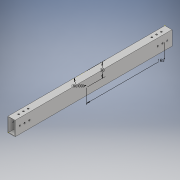
# Autodesk Inventor part: nhk39
Saved by Autodesk Inventor 2019 (Build 230136000, 136)
## iProperties
Created: 2022-02-27
Part Number: nhk39
Material: 一般
Document SubType Name: Sheet Metal
Designer: yuta
Density: 1 g/cm^3
Sheet Metal Rule: Default_mm
Appearance: 既定
Author: yuta
Autodesk Inventor part; units mm, degrees
ref_plane "YZ Plane" through (0, 0, 0) normal (1, 0, 0) x (0, 1, 0)
ref_plane "XZ Plane" through (0, 0, 0) normal (0, 1, 0) x (-1, 0, 0)
ref_plane "XY Plane" through (0, 0, 0) normal (0, 0, 1) x (1, 0, 0)
sketch "スケッチ1" plane through (0, 0, 0) normal (0, 0, 1) x (1, 0, 0)
  line L0 (0, 0) -> (15, 0)
  line L1 (15, 0) -> (15, 30)
  line L2 (15, 30) -> (0, 30)
  line L3 (0, 30) -> (0, 0)
  line L4 (1, 1) -> (14, 1)
  line L5 (14, 1) -> (14, 29)
  line L6 (14, 29) -> (1, 29)
  line L7 (1, 29) -> (1, 1)
  dimension "d0" = 15
  dimension "d1" = 30
  dimension "d2" = 13
  dimension "d3" = 28
  dimension "d4" = 1
  dimension "d5" = 1
  constraints: 16 end point, 4 parallel, 2 horizontal, 2 perpendicular
  measures "d0" distance of L2.end L1.end
  measures "d1" distance of L1.end L0.end
  measures "d2" distance of L6.end L5.end
  measures "d3" distance of L5.end L4.end
  measures "d4" distance between parallel lines of L2 L6
  measures "d5" distance between parallel lines of L3 L7
extrude "押し出し1" add sketch "スケッチ1" along normal blind 330
sketch "スケッチ2" plane through (0, 30, 0) normal (0, 1, 0) x (1, 0, 0)
  circle A0 centre (7.5, -15) radius 1.6
  line L0 (0, 0) -> (0, -330) projected
  line L1 (15, 0) -> (0, 0) projected
  circle A1 centre (7.5, -25) radius 1.6
  circle A2 centre (7.5, -35) radius 1.6
  circle A3 centre (7.5, -315) radius 1.6
  line L2 (15, -330) -> (0, -330) projected
  circle A4 centre (7.5, -305) radius 1.6
  circle A5 centre (7.5, -295) radius 1.6
  dimension "d8" = 3.2
  dimension "d9" = 7.5
  dimension "d10" = 15
  dimension "d11" = 3.2
  dimension "d12" = 10
  dimension "d13" = 3.2
  dimension "d14" = 10
  dimension "d15" = 3.2
  dimension "d16" = 15
  dimension "d17" = 7.5
  dimension "d18" = 3.2
  dimension "d19" = 10
  dimension "d20" = 3.2
  dimension "d21" = 10
  constraints: 6 centre point
  measures "d8" diameter of A0
  measures "d9" distance from line of L0 A0.centre
  measures "d10" distance from line of L1 A0.centre
  measures "d11" diameter of A1
  measures "d12" distance of A0.centre A1.centre
  measures "d13" diameter of A2
  measures "d14" distance of A2.centre A1.centre
  measures "d15" diameter of A3
  measures "d16" distance from line of L2 A3.centre
  measures "d17" distance from line of L0 A3.centre
  measures "d18" diameter of A4
  measures "d19" distance of A3.centre A4.centre
  measures "d20" diameter of A5
  measures "d21" distance of A4.centre A5.centre
hole "穴1" at (7.5, 30, 315) at (7.5, 30, 305) at (7.5, 30, 295) at (7.5, 30, 15) at (7.5, 30, 25) at (7.5, 30, 35) direction (0, -1, 0) diameter 3.2 depth 30
sketch "スケッチ3" plane through (0, 0, 0) normal (-1, 0, 0) x (0, 0, 1)
  circle A0 centre (10, 15) radius 1.6
  line L0 (0, 0) -> (330, 0) projected
  line L1 (0, 30) -> (0, 0) projected
  circle A1 centre (20, 15) radius 1.6
  circle A2 centre (30, 15) radius 1.6
  circle A3 centre (320, 15) radius 1.6
  line L2 (330, 30) -> (330, 0) projected
  circle A4 centre (310, 15) radius 1.6
  circle A5 centre (300, 15) radius 1.6
  dimension "d29" = 3.2
  dimension "d30" = 15
  dimension "d31" = 10
  dimension "d32" = 3.2
  dimension "d33" = 3.2
  dimension "d34" = 10
  dimension "d35" = 10
  dimension "d36" = 3.2
  dimension "d37" = 15
  dimension "d38" = 10
  dimension "d39" = 3.2
  dimension "d40" = 3.2
  dimension "d41" = 10
  dimension "d42" = 10
  dimension "d43" = 15
  dimension "d44" = 15
  dimension "d45" = 15
  dimension "d46" = 15
  constraints: 6 centre point
  measures "d29" diameter of A0
  measures "d30" distance from line of L0 A0.centre
  measures "d31" distance from line of L1 A0.centre
  measures "d32" diameter of A1
  measures "d33" diameter of A2
  measures "d34" distance of A0.centre A1.centre
  measures "d35" distance of A1.centre A2.centre
  measures "d36" diameter of A3
  measures "d37" distance from line of L0 A3.centre
  measures "d38" distance from line of L2 A3.centre
  measures "d39" diameter of A4
  measures "d40" diameter of A5
  measures "d41" distance of A4.centre A3.centre
  measures "d42" distance of A5.centre A4.centre
  measures "d43" distance from line of L0 A4.centre
  measures "d44" distance from line of L0 A5.centre
  measures "d45" distance from line of L0 A1.centre
  measures "d46" distance from line of L0 A2.centre
hole "穴2" at (0, 15, 10) at (0, 15, 20) at (0, 15, 30) at (0, 15, 300) at (0, 15, 310) at (0, 15, 320) direction (1, 0, 0) diameter 3.2 depth 15
sketch "スケッチ4" plane through (0, 0, 0) normal (-1, 0, 0) x (0, 0, 1)
  line L0 (165, 29.8281) -> (165, -0.1719) construction
  line L1 (0, 1) -> (330, 1) projected
  line L2 (165, 29.8281) -> (195, 29.8281) construction
  line L3 (0, 30) -> (0, 0) projected
  dimension "d54" = 30
  dimension "d55" = 90
  dimension "d56" = 165
  constraints: 4 end point, 2 perpendicular, 1 horizontal
  measures "d54" distance of L0.start L0.end
  measures "d55" angle of L0 L2
  measures "d56" distance between parallel lines of L3 L0
sketch "スケッチ5" plane through (0, 0, 0) normal (-1, 0, 0) x (0, 0, 1)
  point P0 (0, 0)
equation "\"BendRadius\" = Thickness"
equation "\"BendReliefWidth\" = Thickness"
equation "\"BendReliefDepth\" = 0.5 * Thickness"
equation "\"CornerReliefSize\" = 4 * Thickness"
equation "\"MinimumRemnant\" = 2 * Thickness"
equation "\"TransitionRadius\" = BendRadius"
equation "\"JacobiRadiusSize\" = BendRadius"
equation "\"GapSize\" = Thickness"
equation "\"Thickness\" = 0.5"
